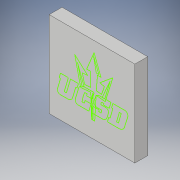
# Autodesk Inventor part: ucsd
Saved by Autodesk Inventor 2018 (Build 220112000, 112)
## iProperties
Created: 2019-04-30
Part Number: ucsd
Material: Generic
Document SubType Name: Modeling
Designer: F8PLTW
Density: 1 g/cm^3
Appearance: Default
Author: F8PLTW
Autodesk Inventor part; units mm, degrees
ref_plane "YZ Plane" through (0, 0, 0) normal (1, 0, 0) x (0, 1, 0)
ref_plane "XZ Plane" through (0, 0, 0) normal (0, 1, 0) x (-1, 0, 0)
ref_plane "XY Plane" through (0, 0, 0) normal (0, 0, 1) x (1, 0, 0)
sketch "Sketch1" plane through (0, 0, 0) normal (0, 0, 1) x (1, 0, 0)
  line L0 (-11.779, 10.0622) -> (39.021, 10.0622)
  line L1 (39.021, 10.0622) -> (39.021, -40.7378)
  line L2 (39.021, -40.7378) -> (-11.779, -40.7378)
  line L3 (-11.779, -40.7378) -> (-11.779, 10.0622)
  point P0 (0, 0)
  dimension "d0" = 50.8
  dimension "d1" = 50.8
  constraints: 8 end point, 2 parallel, 1 horizontal, 1 perpendicular
  measures "d0" distance of L1.end L2.end
  measures "d1" distance of L0.end L1.end
extrude "Extrusion1" add sketch "Sketch1" along normal blind 7.62
sketch "Sketch2" plane through (0, 0, 7.62) normal (0, 0, 1) x (1, 0, 0)
  line L0 (-13.2583, 12.4826) -> (41.5133, 12.4826) construction
  line L1 (41.5133, 12.4826) -> (41.5133, -42.289) construction
  line L2 (41.5133, -42.289) -> (-13.2583, -42.289) construction
  line L3 (-13.2583, -42.289) -> (-13.2583, 12.4826) construction
  point P0 (0, 0)
  constraints: 2 other
sketch "Sketch3" plane through (0, 0, 7.62) normal (0, 0, 1) x (1, 0, 0)
  line L0 (3.3033, -2.76) -> (10.9966, -9.7144)
  line L1 (10.9966, -9.7144) -> (7.8237, -9.9318)
  line L2 (7.8237, -9.9318) -> (9.1277, -15.191)
  line L3 (9.1277, -15.191) -> (12.7391, -14.9437)
  line L4 (12.7391, -14.9437) -> (12.5179, -6.7153)
  line L5 (12.5179, -6.7153) -> (10.3613, -6.7153)
  line L6 (10.3613, -6.7153) -> (14.7781, 3.8901)
  line L7 (3.3033, -2.76) -> (6.8013, -17.9532)
  line L8 (12.7769, -17.3762) -> (13.2763, -31.0832)
  line L9 (13.2763, -31.0832) -> (15.1402, -31.0832)
  line L10 (15.1402, -31.0832) -> (15.9415, -17.3762)
  line L11 (14.7781, 3.8901) -> (18.8649, -6.7153)
  line L12 (18.8649, -6.7153) -> (16.7409, -6.7153)
  line L13 (16.7409, -6.7153) -> (16.0838, -14.9437)
  line L14 (16.0838, -14.9437) -> (19.1698, -15.3512)
  line L15 (20.8744, -10.5043) -> (19.1698, -15.3512)
  line L16 (18.2, -9.8231) -> (20.8744, -10.5043)
  line L17 (25.8628, -3.4744) -> (18.2, -9.8231)
  line L18 (25.8628, -3.4744) -> (21.3619, -17.9532)
  line L19 (21.3619, -17.9532) -> (15.9415, -17.3762)
  line L20 (16.0838, -5.9261) -> (17.6268, -5.9261)
  line L21 (12.7769, -17.3762) -> (6.8013, -17.9532)
  line L22 (14.3821, 2.2995) -> (17.6268, -5.9261)
  line L23 (16.0838, -5.9261) -> (14.3821, 2.2995)
  line L24 (8.8853, -16.6252) -> (4.9497, -5.9874)
  line L25 (4.9497, -5.9874) -> (7.6307, -16.8904)
  line L26 (7.6307, -16.8904) -> (8.8853, -16.6252)
  line L27 (24.2962, -5.9261) -> (21.1437, -16.5685)
  line L28 (24.2962, -5.9261) -> (19.5372, -16.7287)
  line L29 (19.5372, -16.7287) -> (21.1437, -16.5685)
  line L30 (-5.1538, -16.5685) -> (-0.8898, -16.5685)
  line L31 (-2.9354, -24.9367) -> (-0.6239, -17.1332)
  line L32 (-1.6502, -24.9367) -> (-2.9354, -24.9367)
  line L33 (-1.6502, -24.9367) -> (0.7984, -16.6252)
  line L34 (0.7984, -16.6252) -> (5.3544, -16.6252)
  line L35 (4.6604, -19.3073) -> (3.8764, -19.3073)
  line L36 (3.8764, -19.3073) -> (1.8479, -26.1553)
  line L37 (-0.6239, -27.669) -> (-5.3427, -27.669)
  line L38 (-5.1538, -16.5685) -> (-5.7593, -18.6813)
  line L39 (-5.7593, -19.3073) -> (-5.1538, -19.3073)
  line L40 (-5.1538, -19.3073) -> (-6.8493, -25.2235)
  line L41 (4.6604, -19.3073) -> (5.3544, -17.0049)
  line L42 (11.6026, -27.669) -> (5.0523, -27.669)
  line L43 (3.6034, -25.5502) -> (5.6546, -18.6813)
  line L44 (13.6187, -20.402) -> (14.7082, -16.9733)
  line L45 (8.4293, -16.5767) -> (14.3821, -16.5767)
  line L46 (7.6301, -24.9367) -> (8.9504, -24.9367)
  line L47 (8.9504, -24.9367) -> (9.4671, -23.2745)
  line L48 (9.4671, -23.2745) -> (12.7762, -23.2745)
  line L49 (11.6852, -27.5813) -> (12.8623, -23.6074)
  line L50 (10.5482, -20.443) -> (13.4991, -20.443)
  line L51 (10.6116, -19.3074) -> (10.4265, -20.0343)
  line L52 (10.6116, -19.3074) -> (9.2088, -19.3074)
  line L53 (23.7685, -20.1664) -> (24.7257, -16.6252)
  line L54 (24.7257, -16.6252) -> (18.1495, -16.6252)
  line L55 (23.7685, -20.1664) -> (20.4445, -20.1664)
  line L56 (20.4445, -19.788) -> (20.6057, -19.3073)
  line L57 (19.3355, -19.3073) -> (20.4445, -19.3073)
  line L58 (18.7576, -20.6119) -> (19.0513, -19.3897)
  line L59 (18.7576, -20.7809) -> (21.9167, -20.7809)
  line L60 (19.2451, -23.3802) -> (16.4169, -23.3802)
  line L61 (18.9049, -24.9615) -> (17.5187, -24.9615)
  line L62 (17.5187, -24.9615) -> (17.6703, -24.0985)
  line L63 (17.5187, -23.9755) -> (14.2082, -23.9755)
  line L64 (18.9049, -24.9615) -> (19.3355, -23.4656)
  line L65 (20.071, -27.669) -> (13.2254, -27.669)
  line L66 (23.361, -22.5548) -> (22.2655, -26.1891)
  line L67 (25.876, -16.6325) -> (33.2083, -16.6325)
  line L68 (22.9553, -27.6691) -> (29.6245, -27.6691)
  line L69 (34.7748, -18.8891) -> (32.6282, -25.7944)
  line L70 (29.723, -19.3073) -> (30.8661, -19.3073)
  line L71 (30.8661, -19.3073) -> (29.2011, -24.9615)
  line L72 (29.2011, -24.9615) -> (28.0579, -24.9615)
  line L73 (28.0579, -24.9615) -> (29.723, -19.3073)
  line L74 (25.876, -16.6325) -> (25.2006, -18.9262)
  line L75 (25.876, -19.2035) -> (25.2006, -19.2035)
  line L76 (24.2471, -24.9615) -> (25.876, -19.2035)
  line L77 (22.8132, -27.1047) -> (23.4233, -24.9615)
  line L78 (23.4233, -24.9615) -> (24.2471, -24.9615)
  arc A0 (25.2006, -18.9262) -> (25.2006, -19.2035) centre (25.6699, -19.0649) ccw
  arc A1 (34.7748, -18.8891) -> (33.2083, -16.6325) centre (32.8941, -18.5226) ccw
  arc A2 (29.6245, -27.6691) -> (32.6282, -25.7944) centre (29.6245, -24.3253) ccw
  arc A3 (22.8132, -27.1047) -> (22.9553, -27.6691) centre (23.3729, -27.2639) ccw
  arc A4 (20.071, -27.669) -> (22.2655, -26.1891) centre (19.4137, -24.3273) ccw
  arc A5 (23.361, -22.5548) -> (21.9167, -20.7809) centre (21.7369, -22.4023) ccw
  arc A6 (18.7576, -20.6119) -> (18.7576, -20.7809) centre (19.0891, -20.6964) ccw
  arc A7 (19.3355, -19.3073) -> (19.0513, -19.3897) centre (19.3425, -19.8629) ccw
  line L79 (20.6057, -19.3073) -> (20.4445, -19.3073)
  arc A8 (20.4445, -19.788) -> (20.4445, -20.1664) centre (21.2331, -19.9772) ccw
  line L80 (15.8635, -17.7794) -> (14.7323, -20.9077)
  arc A9 (18.1495, -16.6252) -> (15.8635, -17.7794) centre (17.9943, -19.1589) ccw
  arc A10 (14.7323, -20.9077) -> (16.4169, -23.3802) centre (16.4679, -21.5353) ccw
  line L81 (14.2082, -23.9755) -> (13.133, -27.1509)
  arc A11 (13.133, -27.1509) -> (13.2254, -27.669) centre (13.7173, -27.314) ccw
  arc A12 (3.6034, -25.5502) -> (5.0523, -27.669) centre (5.288, -25.953) ccw
  arc A13 (9.2088, -19.3074) -> (7.6301, -24.9367) centre (27.6318, -27.5099) ccw
  arc A14 (8.4293, -16.5767) -> (5.6546, -18.6813) centre (9.3374, -20.6554) ccw
  arc A15 (14.7038, -16.9872) -> (14.3821, -16.5767) centre (14.3663, -16.9203) ccw
  arc A16 (13.4991, -20.443) -> (13.6187, -20.402) centre (13.4991, -20.248) ccw
  arc A17 (10.4265, -20.0343) -> (10.5482, -20.443) centre (10.8291, -20.1368) ccw
  arc A18 (12.8623, -23.6074) -> (12.7762, -23.2745) centre (12.5836, -23.5019) ccw
  arc A19 (-0.6239, -27.669) -> (1.8479, -26.1553) centre (-1.1207, -24.0827) ccw
  arc A20 (-6.8493, -25.2235) -> (-5.3427, -27.669) centre (-5.2757, -25.9409) ccw
  arc A21 (-5.7593, -18.6813) -> (-5.7593, -19.3073) centre (-4.6724, -18.9943) ccw
  arc A22 (-0.6239, -17.1332) -> (-0.8898, -16.5685) centre (-1.0156, -16.9727) ccw
  arc A23 (5.3544, -17.0049) -> (5.3544, -16.6252) centre (4.9273, -16.8151) ccw
  line L82 (14.0136, -30.6187) -> (14.0136, -17.2405)
  line L83 (14.0136, -17.2405) -> (13.3706, -20.1664)
  line L84 (13.3706, -20.1664) -> (13.5921, -30.6322)
  line L85 (13.5921, -30.6322) -> (14.0136, -30.6322)
  line L86 (14.0136, -30.6322) -> (14.0136, -30.6187)
  point P0 (0, 0)
  constraints: 174 end point, 48 point on circle, 29 horizontal, 24 centre point, 5 parallel, 4 point on line, 4 tangent, 1 perpendicular
body "Solid1"
